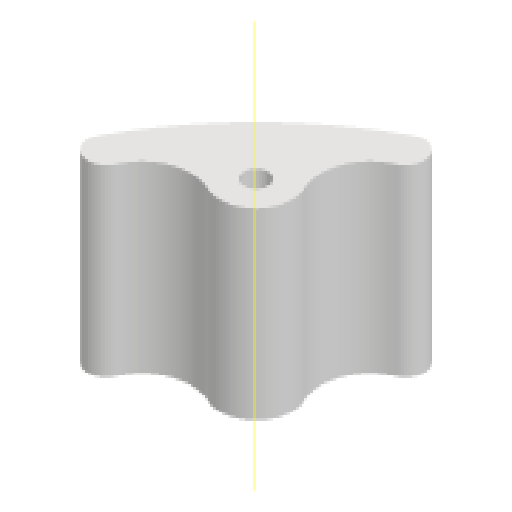
# Autodesk Inventor part: Foam Attachment
Saved by Autodesk Inventor 2025.2 (Build 292293000, 293)
## iProperties
Created: 2025-02-10
Part Number: Foam Attachment
Material: Generic
Document SubType Name: Modeling
Designer: Authorised User
Density: 1 g/cm^3
Appearance: Default
Author: Authorised User
Autodesk Inventor part; units mm, degrees
ref_plane "XZ Plane" through (0, 0, 0) normal (0, 1, 0) x (-1, 0, 0)
ref_plane "XY Plane" through (0, 0, 0) normal (0, 0, 1) x (1, 0, 0)
sketch "Sketch1" plane through (0, 0, 0) normal (0, 1, 0) x (-1, 0, 0)
  arc A0 (31.2876, -56.9744) -> (58.4216, -28.4941) centre (0, 0) ccw
  line L0 (0, -76.4247) -> (0, 75.7077)
  line L1 (75.2776, 0) -> (-75.7077, 0)
  line L2 (0, 0) -> (78.1118, -78.1118)
  line L3 (0, 0) -> (84.1598, -41.0475)
  line L4 (0, 0) -> (41.0475, -84.1598)
  circle A1 centre (38.0152, -38.0152) radius 2
  arc A2 (40.7893, -32.7712) -> (32.7712, -40.7893) centre (38.0152, -38.0152) ccw
  line L5 (27.1472, -55.66) -> (27.0904, -55.5436)
  arc A3 (27.1472, -55.66) -> (31.2876, -56.9744) centre (29.8436, -54.3448) ccw
  arc A4 (28.4686, -51.5336) -> (27.0904, -55.5436) centre (29.7868, -54.2284) ccw
  arc A5 (28.4686, -51.5336) -> (29.2312, -51.1337) centre (-5.4867, 14.1516) ccw
  line L6 (32.7449, -40.7314) -> (32.4923, -40.1813)
  arc A6 (29.2312, -51.1337) -> (32.7449, -40.7314) centre (25.475, -44.0703) ccw
  line L7 (55.66, -27.1472) -> (55.5436, -27.0904)
  arc A7 (56.9744, -31.2876) -> (55.66, -27.1472) centre (54.3448, -29.8436) ccw
  arc A8 (55.5436, -27.0904) -> (51.5336, -28.4686) centre (54.2284, -29.7868) ccw
  arc A9 (51.1337, -29.2312) -> (51.5336, -28.4686) centre (-14.1516, 5.4867) ccw
  arc A10 (40.7314, -32.7449) -> (51.1337, -29.2312) centre (44.0703, -25.475) ccw
  point P0 (28.4941, -58.4216)
  point P1 (25.6079, -52.5039)
  point P2 (35.7325, -47.2364)
  point P3 (55.5436, -27.0904)
  dimension "d0" = 65
  dimension "d1" = 45
  dimension "d2" = 26
  dimension "d3" = 4
  dimension "d4" = 3
  dimension "d6" = 8
  constraints: 25 point on circle, 16 end point, 11 centre point, 11 symmetric about line, 7 point on line, 5 tangent, 2 coincident, 1 equal radius, 1 horizontal, 1 vertical, 4 other
  measures "d0" radius of A0
  measures "d1" angle of L1 L2
  measures "d2" angle of L1 L3
  measures "d3" diameter of A1
  measures "d4" radius of A3
  measures "d6" radius of A6
extrude "Extrusion1" add sketch "Sketch1" along normal blind 30 contours A0 L2 A1 A2 A10 A9 A8 L3 A7 | A0 A3 L4 A4 A5 A6 L6 A2 L2 A1
ref_plane "Work Plane1" through (0, 0, 0) normal (0.7071, 0, -0.7071) x (0, 1, 0)
body "Solid1"
